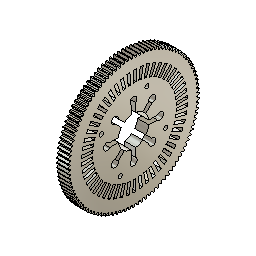
Колесо шестерня v2 (Autodesk Fusion 360 design; units mm, degrees)
Autodesk Fusion 360 part; units mm, degrees
(part 1 of 5)
sketch "Sketch1" plane through (0, 0, 0) normal (1, 0, 0) x (0, 1, 0)
  spline S0 degree 5 poles (13.1929, -43.7407) (13.1941, -43.7421) (13.2057, -43.7558) (13.2278, -43.7819) (13.2606, -43.8203) (13.3041, -43.871) (13.3573, -43.9325) (13.4109, -43.9938) (13.4647, -44.055) (13.5189, -44.116) (13.5735, -44.1768) (13.6283, -44.2375) (13.6834, -44.298) (13.7389, -44.3583) (13.7946, -44.4185) (13.8506, -44.4785) (13.907, -44.5383) (13.9636, -44.5979) (14.0206, -44.6574) (14.0778, -44.7168) (14.1353, -44.7759) (14.1931, -44.8349) (14.2396, -44.882) (14.2745, -44.9172) (14.2979, -44.9406) (14.3096, -44.9524) knots 0.712736 0.712736 0.712736 0.712736 0.712736 0.712736 0.714286 0.728571 0.742857 0.757143 0.771429 0.785714 0.8 0.814286 0.828571 0.842857 0.857143 0.871429 0.885714 0.9 0.914286 0.928571 0.942857 0.957143 0.971429 0.985714 1 1 1 1 1 1
  arc A0 (8.9575, -37.2151) -> (11.0181, -36.7013) centre (0.7975, -0.1016) ccw
  spline S1 degree 5 poles (18.5711, -41.7423) (18.5724, -41.7435) (18.5856, -41.7557) (18.6109, -41.7788) (18.6481, -41.8128) (18.6976, -41.8576) (18.7582, -41.912) (18.819, -41.9661) (18.8801, -42.02) (18.9415, -42.0738) (19.0032, -42.1273) (19.0652, -42.1806) (19.1275, -42.2337) (19.1901, -42.2866) (19.2529, -42.3393) (19.3161, -42.3918) (19.3794, -42.4441) (19.4431, -42.4962) (19.5071, -42.5481) (19.5713, -42.5997) (19.6357, -42.6512) (19.7005, -42.7025) (19.7525, -42.7434) (19.7916, -42.7739) (19.8177, -42.7943) (19.8308, -42.8044) knots 0.712736 0.712736 0.712736 0.712736 0.712736 0.712736 0.714286 0.728571 0.742857 0.757143 0.771429 0.785714 0.8 0.814286 0.828571 0.842857 0.857143 0.871429 0.885714 0.9 0.914286 0.928571 0.942857 0.957143 0.971429 0.985714 1 1 1 1 1 1
  spline S2 degree 5 poles (10.4204, -44.4828) (10.4215, -44.4842) (10.4322, -44.4987) (10.4526, -44.5261) (10.4829, -44.5665) (10.5231, -44.6198) (10.5724, -44.6845) (10.622, -44.7491) (10.6719, -44.8135) (10.7222, -44.8778) (10.7728, -44.9419) (10.8237, -45.0059) (10.8749, -45.0698) (10.9265, -45.1334) (10.9783, -45.197) (11.0305, -45.2604) (11.083, -45.3236) (11.1357, -45.3867) (11.1888, -45.4497) (11.2422, -45.5125) (11.2959, -45.5751) (11.3499, -45.6376) (11.3933, -45.6875) (11.426, -45.7249) (11.4479, -45.7497) (11.4588, -45.7622) knots 0.712736 0.712736 0.712736 0.712736 0.712736 0.712736 0.714286 0.728571 0.742857 0.757143 0.771429 0.785714 0.8 0.814286 0.828571 0.842857 0.857143 0.871429 0.885714 0.9 0.914286 0.928571 0.942857 0.957143 0.971429 0.985714 1 1 1 1 1 1
  spline S3 degree 3 poles (15.9134, -42.826) (15.8674, -42.7781) (15.8125, -42.7397) (15.6911, -42.6859) (15.6257, -42.6712) (15.4929, -42.6676) (15.4268, -42.6788) (15.3026, -42.7258) (15.2457, -42.7613) (15.1487, -42.852) (15.1095, -42.9064) (15.0565, -43.0219) (15.0413, -43.0811) (15.0368, -43.1416) knots 0 0 0 0 0.019923 0.019923 0.039846 0.039846 0.059769 0.059769 0.079691 0.079691 0.099614 0.099614 0.117812 0.117812 0.117812 0.117812
  spline S4 degree 3 poles (13.1929, -43.7407) (13.1501, -43.69) (13.0977, -43.6482) (12.9798, -43.5869) (12.9155, -43.5681) (12.7832, -43.5562) (12.7165, -43.5632) (12.5896, -43.6024) (12.5306, -43.6342) (12.4281, -43.7186) (12.3855, -43.7704) (12.3255, -43.8824) (12.3066, -43.9406) (12.2983, -44.0007) knots 0 0 0 0 0.019923 0.019923 0.039846 0.039846 0.059769 0.059769 0.079691 0.079691 0.099614 0.099614 0.117812 0.117812 0.117812 0.117812
  circle A1 centre (0, 0) radius 11
  circle A2 centre (0, 0) radius 1.5
  spline S5 degree 3 poles (-0.9694, -45.6768) (-0.9945, -45.6153) (-1.0314, -45.5593) (-1.1246, -45.4646) (-1.1799, -45.4268) (-1.3021, -45.3746) (-1.3676, -45.3607) (-1.5004, -45.3587) (-1.5664, -45.3707) (-1.69, -45.4194) (-1.7465, -45.4555) (-1.8382, -45.5434) (-1.8742, -45.5929) (-1.9006, -45.6475) knots 0 0 0 0 0.019923 0.019923 0.039846 0.039846 0.059769 0.059769 0.079691 0.079691 0.099614 0.099614 0.117812 0.117812 0.117812 0.117812
  arc A3 (-0.2495, -30.0833) -> (1.595, -30.091) centre (0.7975, -0.1016) ccw
  spline S6 degree 5 poles (15.9134, -42.826) (15.9146, -42.8273) (15.9271, -42.8403) (15.9508, -42.8649) (15.9859, -42.9012) (16.0325, -42.9491) (16.0895, -43.0071) (16.1468, -43.065) (16.2044, -43.1226) (16.2623, -43.1801) (16.3206, -43.2374) (16.3791, -43.2945) (16.4379, -43.3514) (16.497, -43.4081) (16.5564, -43.4646) (16.6161, -43.521) (16.6761, -43.5772) (16.7364, -43.6332) (16.7969, -43.689) (16.8578, -43.7446) (16.9189, -43.8) (16.9803, -43.8553) (17.0296, -43.8993) (17.0668, -43.9323) (17.0916, -43.9542) (17.104, -43.9652) knots 0.712736 0.712736 0.712736 0.712736 0.712736 0.712736 0.714286 0.728571 0.742857 0.757143 0.771429 0.785714 0.8 0.814286 0.828571 0.842857 0.857143 0.871429 0.885714 0.9 0.914286 0.928571 0.942857 0.957143 0.971429 0.985714 1 1 1 1 1 1
  arc A4 (17.104, -43.9652) -> (17.628, -43.7577) centre (0, 0) ccw
  spline S7 degree 5 poles (17.628, -43.7577) (17.6295, -43.7412) (17.6326, -43.7082) (17.6371, -43.6588) (17.6429, -43.5929) (17.6498, -43.5106) (17.6564, -43.4284) (17.6627, -43.3462) (17.6686, -43.264) (17.6743, -43.182) (17.6795, -43.1) (17.6845, -43.018) (17.6891, -42.9361) (17.6933, -42.8543) (17.6973, -42.7726) (17.7008, -42.6909) (17.7041, -42.6093) (17.707, -42.5277) (17.7095, -42.4462) (17.7117, -42.3648) (17.7135, -42.2835) (17.7147, -42.2168) (17.7154, -42.1663) (17.7158, -42.1321) (17.716, -42.1141) (17.7161, -42.1123) knots -1 -1 -1 -1 -1 -1 -0.985714 -0.971429 -0.957143 -0.942857 -0.928571 -0.914286 -0.9 -0.885714 -0.871429 -0.857143 -0.842857 -0.828571 -0.814286 -0.8 -0.785714 -0.771429 -0.757143 -0.742857 -0.728571 -0.714286 -0.712736 -0.712736 -0.712736 -0.712736 -0.712736 -0.712736
  arc A5 (14.3096, -44.9524) -> (14.8456, -44.7782) centre (0, 0) ccw
  spline S8 degree 5 poles (12.0047, -45.622) (12.0083, -45.6059) (12.0154, -45.5735) (12.0261, -45.525) (12.0401, -45.4604) (12.0573, -45.3796) (12.0742, -45.2989) (12.0907, -45.2181) (12.1069, -45.1374) (12.1228, -45.0566) (12.1383, -44.9759) (12.1534, -44.8953) (12.1683, -44.8146) (12.1828, -44.734) (12.1969, -44.6533) (12.2107, -44.5727) (12.2241, -44.4922) (12.2372, -44.4116) (12.2499, -44.3311) (12.2623, -44.2506) (12.2743, -44.1702) (12.2838, -44.1041) (12.2909, -44.0541) (12.2956, -44.0202) (12.2981, -44.0024) (12.2983, -44.0007) knots -1 -1 -1 -1 -1 -1 -0.985714 -0.971429 -0.957143 -0.942857 -0.928571 -0.914286 -0.9 -0.885714 -0.871429 -0.857143 -0.842857 -0.828571 -0.814286 -0.8 -0.785714 -0.771429 -0.757143 -0.742857 -0.728571 -0.714286 -0.712736 -0.712736 -0.712736 -0.712736 -0.712736 -0.712736
  spline S9 degree 5 poles (14.8456, -44.7782) (14.8482, -44.7619) (14.8533, -44.7291) (14.8609, -44.6801) (14.8709, -44.6147) (14.8829, -44.533) (14.8947, -44.4513) (14.9061, -44.3697) (14.9172, -44.2881) (14.928, -44.2065) (14.9384, -44.125) (14.9485, -44.0436) (14.9582, -43.9621) (14.9676, -43.8807) (14.9766, -43.7994) (14.9853, -43.7181) (14.9937, -43.6368) (15.0017, -43.5556) (15.0093, -43.4745) (15.0166, -43.3934) (15.0235, -43.3123) (15.0289, -43.2458) (15.0328, -43.1954) (15.0354, -43.1613) (15.0367, -43.1434) (15.0368, -43.1416) knots -1 -1 -1 -1 -1 -1 -0.985714 -0.971429 -0.957143 -0.942857 -0.928571 -0.914286 -0.9 -0.885714 -0.871429 -0.857143 -0.842857 -0.828571 -0.814286 -0.8 -0.785714 -0.771429 -0.757143 -0.742857 -0.728571 -0.714286 -0.712736 -0.712736 -0.712736 -0.712736 -0.712736 -0.712736
  spline S10 degree 5 poles (21.1555, -40.4939) (21.1568, -40.495) (21.1708, -40.5063) (21.1974, -40.5278) (21.2368, -40.5594) (21.289, -40.601) (21.3528, -40.6514) (21.4169, -40.7016) (21.4813, -40.7516) (21.546, -40.8014) (21.6109, -40.8509) (21.6762, -40.9002) (21.7417, -40.9493) (21.8074, -40.9982) (21.8734, -41.0468) (21.9397, -41.0953) (22.0063, -41.1435) (22.0731, -41.1915) (22.1402, -41.2392) (22.2075, -41.2868) (22.2751, -41.3341) (22.3429, -41.3812) (22.3974, -41.4188) (22.4383, -41.4468) (22.4657, -41.4655) (22.4794, -41.4748) knots 0.712736 0.712736 0.712736 0.712736 0.712736 0.712736 0.714286 0.728571 0.742857 0.757143 0.771429 0.785714 0.8 0.814286 0.828571 0.842857 0.857143 0.871429 0.885714 0.9 0.914286 0.928571 0.942857 0.957143 0.971429 0.985714 1 1 1 1 1 1
  spline S11 degree 3 poles (21.1555, -40.4939) (21.1038, -40.4521) (21.0445, -40.4208) (20.9173, -40.3827) (20.8506, -40.3763) (20.7184, -40.3894) (20.6542, -40.4087) (20.5369, -40.471) (20.4849, -40.5133) (20.4, -40.6155) (20.3679, -40.6743) (20.3299, -40.7956) (20.3222, -40.8562) (20.3254, -40.9168) knots 0 0 0 0 0.019923 0.019923 0.039846 0.039846 0.059769 0.059769 0.079691 0.079691 0.099614 0.099614 0.117812 0.117812 0.117812 0.117812
  spline S12 degree 3 poles (23.6563, -39.0856) (23.6022, -39.0471) (23.541, -39.0196) (23.4117, -38.9896) (23.3447, -38.9874) (23.2136, -39.0087) (23.1507, -39.0321) (23.0376, -39.1016) (22.9883, -39.1471) (22.91, -39.2544) (22.8817, -39.3152) (22.8514, -39.4386) (22.8475, -39.4996) (22.8544, -39.5598) knots 0 0 0 0 0.019923 0.019923 0.039846 0.039846 0.059769 0.059769 0.079691 0.079691 0.099614 0.099614 0.117812 0.117812 0.117812 0.117812
  spline S13 degree 5 poles (22.9733, -41.2033) (22.9727, -41.1867) (22.9716, -41.1536) (22.9699, -41.104) (22.9674, -41.0379) (22.964, -40.9554) (22.9602, -40.873) (22.9561, -40.7907) (22.9517, -40.7084) (22.947, -40.6263) (22.942, -40.5443) (22.9366, -40.4624) (22.9309, -40.3805) (22.9249, -40.2988) (22.9185, -40.2172) (22.9118, -40.1357) (22.9048, -40.0544) (22.8975, -39.9731) (22.8898, -39.892) (22.8817, -39.8109) (22.8733, -39.73) (22.8662, -39.6636) (22.8606, -39.6135) (22.8567, -39.5795) (22.8546, -39.5616) (22.8544, -39.5598) knots -1 -1 -1 -1 -1 -1 -0.985714 -0.971429 -0.957143 -0.942857 -0.928571 -0.914286 -0.9 -0.885714 -0.871429 -0.857143 -0.842857 -0.828571 -0.814286 -0.8 -0.785714 -0.771429 -0.757143 -0.742857 -0.728571 -0.714286 -0.712736 -0.712736 -0.712736 -0.712736 -0.712736 -0.712736
  spline S14 degree 3 poles (18.5711, -41.7423) (18.5222, -41.6974) (18.465, -41.6624) (18.3404, -41.6164) (18.2742, -41.6058) (18.1414, -41.6106) (18.0762, -41.6259) (17.9552, -41.6807) (17.9006, -41.7196) (17.8095, -41.8162) (17.7738, -41.873) (17.7282, -41.9916) (17.7167, -42.0517) (17.7161, -42.1123) knots 0 0 0 0 0.019923 0.019923 0.039846 0.039846 0.059769 0.059769 0.079691 0.079691 0.099614 0.099614 0.117812 0.117812 0.117812 0.117812
  arc A6 (11.4588, -45.7622) -> (12.0047, -45.622) centre (0, 0) ccw
  spline S15 degree 3 poles (4.7631, -45.4381) (4.7304, -45.3802) (4.6868, -45.3293) (4.5825, -45.2471) (4.5229, -45.2165) (4.3952, -45.18) (4.3283, -45.1744) (4.1963, -45.1891) (4.1324, -45.2093) (4.0159, -45.273) (3.9644, -45.316) (3.8844, -45.4147) (3.8549, -45.4683) (3.8356, -45.5258) knots 0 0 0 0 0.019923 0.019923 0.039846 0.039846 0.059769 0.059769 0.079691 0.079691 0.099614 0.099614 0.117812 0.117812 0.117812 0.117812
  spline S16 degree 5 poles (20.3407, -42.5645) (20.3413, -42.5479) (20.3422, -42.5148) (20.3436, -42.4652) (20.3453, -42.3991) (20.347, -42.3165) (20.3485, -42.234) (20.3496, -42.1516) (20.3504, -42.0693) (20.3508, -41.987) (20.3509, -41.9048) (20.3507, -41.8227) (20.3502, -41.7407) (20.3493, -41.6588) (20.3481, -41.5769) (20.3465, -41.4952) (20.3446, -41.4135) (20.3423, -41.332) (20.3398, -41.2505) (20.3368, -41.1691) (20.3335, -41.0878) (20.3305, -41.0211) (20.3281, -40.9707) (20.3264, -40.9365) (20.3254, -40.9186) (20.3254, -40.9168) knots -1 -1 -1 -1 -1 -1 -0.985714 -0.971429 -0.957143 -0.942857 -0.928571 -0.914286 -0.9 -0.885714 -0.871429 -0.857143 -0.842857 -0.828571 -0.814286 -0.8 -0.785714 -0.771429 -0.757143 -0.742857 -0.728571 -0.714286 -0.712736 -0.712736 -0.712736 -0.712736 -0.712736 -0.712736
  arc A7 (4.2415, -37.9452) -> (6.3503, -37.6937) centre (0.7975, -0.1016) ccw
  arc A8 (19.8308, -42.8044) -> (20.3407, -42.5645) centre (0, 0) ccw
  spline S17 degree 5 poles (-0.9694, -45.6768) (-0.9687, -45.6784) (-0.9619, -45.695) (-0.9489, -45.7267) (-0.9297, -45.7734) (-0.904, -45.835) (-0.8723, -45.9099) (-0.8404, -45.9848) (-0.808, -46.0596) (-0.7753, -46.1344) (-0.7423, -46.2091) (-0.7089, -46.2837) (-0.6751, -46.3583) (-0.641, -46.4328) (-0.6066, -46.5072) (-0.5719, -46.5816) (-0.5368, -46.6559) (-0.5013, -46.7302) (-0.4656, -46.8043) (-0.4295, -46.8784) (-0.3931, -46.9525) (-0.3563, -47.0264) (-0.3267, -47.0856) (-0.3043, -47.1299) (-0.2893, -47.1594) (-0.2818, -47.1742) knots 0.712736 0.712736 0.712736 0.712736 0.712736 0.712736 0.714286 0.728571 0.742857 0.757143 0.771429 0.785714 0.8 0.814286 0.828571 0.842857 0.857143 0.871429 0.885714 0.9 0.914286 0.928571 0.942857 0.957143 0.971429 0.985714 1 1 1 1 1 1
  arc A9 (-0.2818, -47.1742) -> (0.2818, -47.1742) centre (0, 0) ccw
  spline S18 degree 3 poles (10.4204, -44.4828) (10.3808, -44.4295) (10.3311, -44.3845) (10.2174, -44.3159) (10.1543, -44.2931) (10.0231, -44.2729) (9.9561, -44.2757) (9.827, -44.3069) (9.7661, -44.3349) (9.6584, -44.4127) (9.6127, -44.4618) (9.5457, -44.5698) (9.5232, -44.6266) (9.5112, -44.686) knots 0 0 0 0 0.019923 0.019923 0.039846 0.039846 0.059769 0.059769 0.079691 0.079691 0.099614 0.099614 0.117812 0.117812 0.117812 0.117812
  spline S19 degree 5 poles (9.1163, -46.2858) (9.121, -46.2699) (9.1301, -46.2381) (9.1438, -46.1903) (9.1619, -46.1267) (9.1841, -46.0472) (9.206, -45.9676) (9.2276, -45.8881) (9.2488, -45.8085) (9.2697, -45.7289) (9.2903, -45.6494) (9.3105, -45.5698) (9.3303, -45.4902) (9.3498, -45.4106) (9.369, -45.3311) (9.3878, -45.2515) (9.4063, -45.1719) (9.4244, -45.0924) (9.4422, -45.0128) (9.4596, -44.9333) (9.4766, -44.8537) (9.4903, -44.7884) (9.5005, -44.7389) (9.5073, -44.7054) (9.5109, -44.6878) (9.5112, -44.686) knots -1 -1 -1 -1 -1 -1 -0.985714 -0.971429 -0.957143 -0.942857 -0.928571 -0.914286 -0.9 -0.885714 -0.871429 -0.857143 -0.842857 -0.828571 -0.814286 -0.8 -0.785714 -0.771429 -0.757143 -0.742857 -0.728571 -0.714286 -0.712736 -0.712736 -0.712736 -0.712736 -0.712736 -0.712736
  spline S20 degree 3 poles (1.9006, -45.6475) (1.8717, -45.5877) (1.8313, -45.5342) (1.7324, -45.4455) (1.6748, -45.4113) (1.5496, -45.3668) (1.4833, -45.3571) (1.3506, -45.3634) (1.2855, -45.3796) (1.1652, -45.4359) (1.1112, -45.4755) (1.0251, -45.569) (0.9923, -45.6206) (0.9694, -45.6768) knots 0 0 0 0 0.019923 0.019923 0.039846 0.039846 0.059769 0.059769 0.079691 0.079691 0.099614 0.099614 0.117812 0.117812 0.117812 0.117812
  arc A10 (2.6809, -47.0988) -> (3.2433, -47.0634) centre (0, 0) ccw
  spline S21 degree 5 poles (7.6067, -45.0493) (7.6077, -45.0508) (7.6175, -45.0659) (7.6362, -45.0946) (7.6639, -45.1368) (7.7007, -45.1925) (7.7458, -45.2602) (7.7912, -45.3278) (7.837, -45.3952) (7.8831, -45.4625) (7.9296, -45.5297) (7.9764, -45.5967) (8.0235, -45.6637) (8.0709, -45.7305) (8.1187, -45.7971) (8.1668, -45.8637) (8.2152, -45.9301) (8.2639, -45.9964) (8.3129, -46.0625) (8.3623, -46.1286) (8.4119, -46.1945) (8.4619, -46.2602) (8.5021, -46.3128) (8.5324, -46.3521) (8.5526, -46.3783) (8.5628, -46.3914) knots 0.712736 0.712736 0.712736 0.712736 0.712736 0.712736 0.714286 0.728571 0.742857 0.757143 0.771429 0.785714 0.8 0.814286 0.828571 0.842857 0.857143 0.871429 0.885714 0.9 0.914286 0.928571 0.942857 0.957143 0.971429 0.985714 1 1 1 1 1 1
  arc A11 (22.4794, -41.4748) -> (22.9733, -41.2033) centre (0, 0) ccw
  spline S22 degree 5 poles (4.7631, -45.4381) (4.7639, -45.4396) (4.7728, -45.4553) (4.7896, -45.4851) (4.8146, -45.5289) (4.8478, -45.5869) (4.8886, -45.6572) (4.9297, -45.7275) (4.9712, -45.7977) (5.013, -45.8678) (5.0551, -45.9377) (5.0976, -46.0076) (5.1404, -46.0774) (5.1836, -46.147) (5.2271, -46.2165) (5.2709, -46.286) (5.315, -46.3553) (5.3595, -46.4245) (5.4042, -46.4936) (5.4493, -46.5626) (5.4947, -46.6315) (5.5405, -46.7003) (5.5773, -46.7552) (5.6051, -46.7964) (5.6236, -46.8238) (5.6329, -46.8375) knots 0.712736 0.712736 0.712736 0.712736 0.712736 0.712736 0.714286 0.728571 0.742857 0.757143 0.771429 0.785714 0.8 0.814286 0.828571 0.842857 0.857143 0.871429 0.885714 0.9 0.914286 0.928571 0.942857 0.957143 0.971429 0.985714 1 1 1 1 1 1
  arc A12 (-0.5287, -38.0785) -> (1.595, -38.0932) centre (0.7975, -0.1016) ccw
  spline S23 degree 3 poles (7.6067, -45.0493) (7.5705, -44.9937) (7.5238, -44.9456) (7.4146, -44.87) (7.3531, -44.8433) (7.2234, -44.8149) (7.1563, -44.8135) (7.0255, -44.8365) (6.963, -44.8606) (6.8507, -44.9315) (6.802, -44.9776) (6.7283, -45.0812) (6.7023, -45.1365) (6.6866, -45.1951) knots 0 0 0 0 0.019923 0.019923 0.039846 0.039846 0.059769 0.059769 0.079691 0.079691 0.099614 0.099614 0.117812 0.117812 0.117812 0.117812
  arc A13 (8.5628, -46.3914) -> (9.1163, -46.2858) centre (0, 0) ccw
  spline S24 degree 5 poles (1.9006, -45.6475) (1.9013, -45.6491) (1.9092, -45.6653) (1.9241, -45.6961) (1.9463, -45.7414) (1.9758, -45.8013) (2.0121, -45.8741) (2.0487, -45.9468) (2.0857, -46.0195) (2.123, -46.092) (2.1607, -46.1645) (2.1987, -46.2369) (2.2371, -46.3092) (2.2758, -46.3814) (2.3148, -46.4536) (2.3542, -46.5256) (2.3938, -46.5976) (2.4339, -46.6694) (2.4742, -46.7412) (2.5149, -46.8129) (2.5559, -46.8845) (2.5972, -46.956) (2.6305, -47.0132) (2.6556, -47.056) (2.6724, -47.0845) (2.6809, -47.0988) knots 0.712736 0.712736 0.712736 0.712736 0.712736 0.712736 0.714286 0.728571 0.742857 0.757143 0.771429 0.785714 0.8 0.814286 0.828571 0.842857 0.857143 0.871429 0.885714 0.9 0.914286 0.928571 0.942857 0.957143 0.971429 0.985714 1 1 1 1 1 1
  spline S25 degree 5 poles (6.192, -46.7669) (6.1976, -46.7513) (6.2088, -46.7201) (6.2255, -46.6733) (6.2475, -46.611) (6.2747, -46.533) (6.3015, -46.455) (6.328, -46.3769) (6.3542, -46.2988) (6.3801, -46.2207) (6.4056, -46.1426) (6.4307, -46.0645) (6.4556, -45.9863) (6.48, -45.9081) (6.5042, -45.8299) (6.5279, -45.7517) (6.5514, -45.6734) (6.5744, -45.5952) (6.5972, -45.5169) (6.6195, -45.4386) (6.6415, -45.3603) (6.6593, -45.2959) (6.6725, -45.2472) (6.6815, -45.2142) (6.6861, -45.1968) (6.6866, -45.1951) knots -1 -1 -1 -1 -1 -1 -0.985714 -0.971429 -0.957143 -0.942857 -0.928571 -0.914286 -0.9 -0.885714 -0.871429 -0.857143 -0.842857 -0.828571 -0.814286 -0.8 -0.785714 -0.771429 -0.757143 -0.742857 -0.728571 -0.714286 -0.712736 -0.712736 -0.712736 -0.712736 -0.712736 -0.712736
  spline S26 degree 3 poles (-1.9006, 45.6475) (-1.8717, 45.5877) (-1.8313, 45.5342) (-1.7324, 45.4455) (-1.6748, 45.4113) (-1.5496, 45.3668) (-1.4833, 45.3571) (-1.3506, 45.3634) (-1.2855, 45.3796) (-1.1652, 45.4359) (-1.1112, 45.4755) (-1.0251, 45.569) (-0.9923, 45.6206) (-0.9694, 45.6768) knots 0 0 0 0 0.019923 0.019923 0.039846 0.039846 0.059769 0.059769 0.079691 0.079691 0.099614 0.099614 0.117812 0.117812 0.117812 0.117812
  arc A14 (5.6329, -46.8375) -> (6.192, -46.7669) centre (0, 0) ccw
  spline S27 degree 5 poles (3.2433, -47.0634) (3.2499, -47.0482) (3.263, -47.0178) (3.2825, -46.9721) (3.3084, -46.9113) (3.3405, -46.8351) (3.3722, -46.759) (3.4035, -46.6827) (3.4346, -46.6065) (3.4653, -46.5301) (3.4956, -46.4538) (3.5256, -46.3774) (3.5553, -46.3009) (3.5847, -46.2244) (3.6137, -46.1479) (3.6423, -46.0713) (3.6706, -45.9947) (3.6985, -45.918) (3.7261, -45.8413) (3.7533, -45.7646) (3.7802, -45.6878) (3.802, -45.6247) (3.8183, -45.5769) (3.8292, -45.5445) (3.835, -45.5274) (3.8356, -45.5258) knots -1 -1 -1 -1 -1 -1 -0.985714 -0.971429 -0.957143 -0.942857 -0.928571 -0.914286 -0.9 -0.885714 -0.871429 -0.857143 -0.842857 -0.828571 -0.814286 -0.8 -0.785714 -0.771429 -0.757143 -0.742857 -0.728571 -0.714286 -0.712736 -0.712736 -0.712736 -0.712736 -0.712736 -0.712736
  spline S28 degree 5 poles (0.2818, -47.1742) (0.2893, -47.1594) (0.3043, -47.1299) (0.3267, -47.0856) (0.3563, -47.0264) (0.3931, -46.9525) (0.4295, -46.8784) (0.4656, -46.8043) (0.5013, -46.7302) (0.5368, -46.6559) (0.5719, -46.5816) (0.6066, -46.5072) (0.641, -46.4328) (0.6751, -46.3583) (0.7089, -46.2837) (0.7423, -46.2091) (0.7753, -46.1344) (0.808, -46.0596) (0.8404, -45.9848) (0.8723, -45.9099) (0.904, -45.835) (0.9297, -45.7734) (0.9489, -45.7267) (0.9619, -45.695) (0.9687, -45.6784) (0.9694, -45.6768) knots -1 -1 -1 -1 -1 -1 -0.985714 -0.971429 -0.957143 -0.942857 -0.928571 -0.914286 -0.9 -0.885714 -0.871429 -0.857143 -0.842857 -0.828571 -0.814286 -0.8 -0.785714 -0.771429 -0.757143 -0.742857 -0.728571 -0.714286 -0.712736 -0.712736 -0.712736 -0.712736 -0.712736 -0.712736
  arc A15 (3.5165, -29.9781) -> (5.3474, -29.7546) centre (0.7975, -0.1016) ccw
  arc A16 (22.0468, -31.605) -> (23.7736, -30.3687) centre (0.7975, -0.1016) ccw
  line L0 (19.07, -23.8948) -> (23.7736, -30.3687)
  spline S29 degree 3 poles (45.1951, -6.6866) (45.1309, -6.7038) (45.0708, -6.7334) (44.9652, -6.8139) (44.9207, -6.8641) (44.8536, -6.9787) (44.8316, -7.0421) (44.813, -7.1736) (44.8167, -7.2405) (44.8494, -7.3692) (44.8782, -7.4298) (44.9539, -7.5318) (44.9985, -7.5737) (45.0493, -7.6067) knots 0 0 0 0 0.019923 0.019923 0.039846 0.039846 0.059769 0.059769 0.079691 0.079691 0.099614 0.099614 0.117812 0.117812 0.117812 0.117812
  spline S30 degree 3 poles (42.1123, -17.7161) (42.0459, -17.7168) (41.9803, -17.7305) (41.858, -17.7822) (41.8024, -17.8198) (41.7089, -17.9141) (41.6718, -17.97) (41.6211, -18.0927) (41.608, -18.1585) (41.6077, -18.2913) (41.6206, -18.3571) (41.6685, -18.4748) (41.7013, -18.5264) (41.7423, -18.5711) knots 0 0 0 0 0.019923 0.019923 0.039846 0.039846 0.059769 0.059769 0.079691 0.079691 0.099614 0.099614 0.117812 0.117812 0.117812 0.117812
  arc A17 (44.7782, -14.8456) -> (44.9524, -14.3096) centre (0, 0) ccw
  spline S31 degree 5 poles (42.1123, -17.7161) (42.1141, -17.716) (42.1321, -17.7158) (42.1663, -17.7154) (42.2168, -17.7147) (42.2835, -17.7135) (42.3648, -17.7117) (42.4462, -17.7095) (42.5277, -17.707) (42.6093, -17.7041) (42.6909, -17.7008) (42.7726, -17.6973) (42.8543, -17.6933) (42.9361, -17.6891) (43.018, -17.6845) (43.1, -17.6795) (43.182, -17.6743) (43.264, -17.6686) (43.3462, -17.6627) (43.4284, -17.6564) (43.5106, -17.6498) (43.5929, -17.6429) (43.6588, -17.6371) (43.7082, -17.6326) (43.7412, -17.6295) (43.7577, -17.628) knots 0.712736 0.712736 0.712736 0.712736 0.712736 0.712736 0.714286 0.728571 0.742857 0.757143 0.771429 0.785714 0.8 0.814286 0.828571 0.842857 0.857143 0.871429 0.885714 0.9 0.914286 0.928571 0.942857 0.957143 0.971429 0.985714 1 1 1 1 1 1
  spline S32 degree 5 poles (45.5258, -3.8356) (45.5274, -3.835) (45.5445, -3.8292) (45.5769, -3.8183) (45.6247, -3.802) (45.6878, -3.7802) (45.7646, -3.7533) (45.8413, -3.7261) (45.918, -3.6985) (45.9947, -3.6706) (46.0713, -3.6423) (46.1479, -3.6137) (46.2244, -3.5847) (46.3009, -3.5553) (46.3774, -3.5256) (46.4538, -3.4956) (46.5301, -3.4653) (46.6065, -3.4346) (46.6827, -3.4035) (46.759, -3.3722) (46.8351, -3.3405) (46.9113, -3.3084) (46.9721, -3.2825) (47.0178, -3.263) (47.0482, -3.2499) (47.0634, -3.2433) knots 0.712736 0.712736 0.712736 0.712736 0.712736 0.712736 0.714286 0.728571 0.742857 0.757143 0.771429 0.785714 0.8 0.814286 0.828571 0.842857 0.857143 0.871429 0.885714 0.9 0.914286 0.928571 0.942857 0.957143 0.971429 0.985714 1 1 1 1 1 1
  arc A18 (46.2858, -9.1163) -> (46.3914, -8.5628) centre (0, 0) ccw
  spline S33 degree 3 poles (43.1416, -15.0368) (43.0754, -15.0417) (43.0107, -15.0595) (42.8919, -15.1189) (42.8389, -15.1599) (42.7515, -15.2599) (42.718, -15.3179) (42.6751, -15.4436) (42.6661, -15.5101) (42.6741, -15.6426) (42.6911, -15.7075) (42.7464, -15.8219) (42.7823, -15.8714) (42.826, -15.9134) knots 0 0 0 0 0.019923 0.019923 0.039846 0.039846 0.059769 0.059769 0.079691 0.079691 0.099614 0.099614 0.117812 0.117812 0.117812 0.117812
  arc A19 (47.0634, -3.2433) -> (47.0988, -2.6809) centre (0, 0) ccw
  spline S34 degree 5 poles (47.0988, -2.6809) (47.0845, -2.6724) (47.056, -2.6556) (47.0132, -2.6305) (46.956, -2.5972) (46.8845, -2.5559) (46.8129, -2.5149) (46.7412, -2.4742) (46.6694, -2.4339) (46.5976, -2.3938) (46.5256, -2.3542) (46.4536, -2.3148) (46.3814, -2.2758) (46.3092, -2.2371) (46.2369, -2.1987) (46.1645, -2.1607) (46.092, -2.123) (46.0195, -2.0857) (45.9468, -2.0487) (45.8741, -2.0121) (45.8013, -1.9758) (45.7414, -1.9463) (45.6961, -1.9241) (45.6653, -1.9092) (45.6491, -1.9013) (45.6475, -1.9006) knots -1 -1 -1 -1 -1 -1 -0.985714 -0.971429 -0.957143 -0.942857 -0.928571 -0.914286 -0.9 -0.885714 -0.871429 -0.857143 -0.842857 -0.828571 -0.814286 -0.8 -0.785714 -0.771429 -0.757143 -0.742857 -0.728571 -0.714286 -0.712736 -0.712736 -0.712736 -0.712736 -0.712736 -0.712736
  spline S35 degree 5 poles (43.9652, -17.104) (43.9542, -17.0916) (43.9323, -17.0668) (43.8993, -17.0296) (43.8553, -16.9803) (43.8, -16.9189) (43.7446, -16.8578) (43.689, -16.7969) (43.6332, -16.7364) (43.5772, -16.6761) (43.521, -16.6161) (43.4646, -16.5564) (43.4081, -16.497) (43.3514, -16.4379) (43.2945, -16.3791) (43.2374, -16.3206) (43.1801, -16.2623) (43.1226, -16.2044) (43.065, -16.1468) (43.0071, -16.0895) (42.9491, -16.0325) (42.9012, -15.9859) (42.8649, -15.9508) (42.8403, -15.9271) (42.8273, -15.9146) (42.826, -15.9134) knots -1 -1 -1 -1 -1 -1 -0.985714 -0.971429 -0.957143 -0.942857 -0.928571 -0.914286 -0.9 -0.885714 -0.871429 -0.857143 -0.842857 -0.828571 -0.814286 -0.8 -0.785714 -0.771429 -0.757143 -0.742857 -0.728571 -0.714286 -0.712736 -0.712736 -0.712736 -0.712736 -0.712736 -0.712736
  spline S36 degree 5 poles (46.8375, -5.6329) (46.8238, -5.6236) (46.7964, -5.6051) (46.7552, -5.5773) (46.7003, -5.5405) (46.6315, -5.4947) (46.5626, -5.4493) (46.4936, -5.4042) (46.4245, -5.3595) (46.3553, -5.315) (46.286, -5.2709) (46.2165, -5.2271) (46.147, -5.1836) (46.0774, -5.1404) (46.0076, -5.0976) (45.9377, -5.0551) (45.8678, -5.013) (45.7977, -4.9712) (45.7275, -4.9297) (45.6572, -4.8886) (45.5869, -4.8478) (45.5289, -4.8146) (45.4851, -4.7896) (45.4553, -4.7728) (45.4396, -4.7639) (45.4381, -4.7631) knots -1 -1 -1 -1 -1 -1 -0.985714 -0.971429 -0.957143 -0.942857 -0.928571 -0.914286 -0.9 -0.885714 -0.871429 -0.857143 -0.842857 -0.828571 -0.814286 -0.8 -0.785714 -0.771429 -0.757143 -0.742857 -0.728571 -0.714286 -0.712736 -0.712736 -0.712736 -0.712736 -0.712736 -0.712736
  arc A20 (46.7669, -6.192) -> (46.8375, -5.6329) centre (0, 0) ccw
  spline S37 degree 5 poles (45.7622, -11.4588) (45.7497, -11.4479) (45.7249, -11.426) (45.6875, -11.3933) (45.6376, -11.3499) (45.5751, -11.2959) (45.5125, -11.2422) (45.4497, -11.1888) (45.3867, -11.1357) (45.3236, -11.083) (45.2604, -11.0305) (45.197, -10.9783) (45.1334, -10.9265) (45.0698, -10.8749) (45.0059, -10.8237) (44.9419, -10.7728) (44.8778, -10.7222) (44.8135, -10.6719) (44.7491, -10.622) (44.6845, -10.5724) (44.6198, -10.5231) (44.5665, -10.4829) (44.5261, -10.4526) (44.4987, -10.4322) (44.4842, -10.4215) (44.4828, -10.4204) knots -1 -1 -1 -1 -1 -1 -0.985714 -0.971429 -0.957143 -0.942857 -0.928571 -0.914286 -0.9 -0.885714 -0.871429 -0.857143 -0.842857 -0.828571 -0.814286 -0.8 -0.785714 -0.771429 -0.757143 -0.742857 -0.728571 -0.714286 -0.712736 -0.712736 -0.712736 -0.712736 -0.712736 -0.712736
  spline S38 degree 5 poles (44.0007, -12.2983) (44.0024, -12.2981) (44.0202, -12.2956) (44.0541, -12.2909) (44.1041, -12.2838) (44.1702, -12.2743) (44.2506, -12.2623) (44.3311, -12.2499) (44.4116, -12.2372) (44.4922, -12.2241) (44.5727, -12.2107) (44.6533, -12.1969) (44.734, -12.1828) (44.8146, -12.1683) (44.8953, -12.1534) (44.9759, -12.1383) (45.0566, -12.1228) (45.1374, -12.1069) (45.2181, -12.0907) (45.2989, -12.0742) (45.3796, -12.0573) (45.4604, -12.0401) (45.525, -12.0261) (45.5735, -12.0154) (45.6059, -12.0083) (45.622, -12.0047) knots 0.712736 0.712736 0.712736 0.712736 0.712736 0.712736 0.714286 0.728571 0.742857 0.757143 0.771429 0.785714 0.8 0.814286 0.828571 0.842857 0.857143 0.871429 0.885714 0.9 0.914286 0.928571 0.942857 0.957143 0.971429 0.985714 1 1 1 1 1 1
  spline S39 degree 5 poles (44.9524, -14.3096) (44.9406, -14.2979) (44.9172, -14.2745) (44.882, -14.2396) (44.8349, -14.1931) (44.7759, -14.1353) (44.7168, -14.0778) (44.6574, -14.0206) (44.5979, -13.9636) (44.5383, -13.907) (44.4785, -13.8506) (44.4185, -13.7946) (44.3583, -13.7389) (44.298, -13.6834) (44.2375, -13.6283) (44.1768, -13.5735) (44.116, -13.5189) (44.055, -13.4647) (43.9938, -13.4109) (43.9325, -13.3573) (43.871, -13.3041) (43.8203, -13.2606) (43.7819, -13.2278) (43.7558, -13.2057) (43.7421, -13.1941) (43.7407, -13.1929) knots -1 -1 -1 -1 -1 -1 -0.985714 -0.971429 -0.957143 -0.942857 -0.928571 -0.914286 -0.9 -0.885714 -0.871429 -0.857143 -0.842857 -0.828571 -0.814286 -0.8 -0.785714 -0.771429 -0.757143 -0.742857 -0.728571 -0.714286 -0.712736 -0.712736 -0.712736 -0.712736 -0.712736 -0.712736
  spline S40 degree 3 poles (45.6768, -0.9694) (45.6153, -0.9945) (45.5593, -1.0314) (45.4646, -1.1246) (45.4268, -1.1799) (45.3746, -1.3021) (45.3607, -1.3676) (45.3587, -1.5004) (45.3707, -1.5664) (45.4194, -1.69) (45.4555, -1.7465) (45.5434, -1.8382) (45.5929, -1.8742) (45.6475, -1.9006) knots 0 0 0 0 0.019923 0.019923 0.039846 0.039846 0.059769 0.059769 0.079691 0.079691 0.099614 0.099614 0.117812 0.117812 0.117812 0.117812
  spline S41 degree 5 poles (23.6563, -39.0856) (23.6578, -39.0866) (23.6724, -39.097) (23.7004, -39.1168) (23.7416, -39.1459) (23.7964, -39.1841) (23.8632, -39.2305) (23.9304, -39.2765) (23.9978, -39.3224) (24.0654, -39.368) (24.1333, -39.4133) (24.2015, -39.4585) (24.27, -39.5033) (24.3387, -39.548) (24.4076, -39.5924) (24.4768, -39.6366) (24.5463, -39.6805) (24.616, -39.7242) (24.6859, -39.7677) (24.7561, -39.8109) (24.8265, -39.8539) (24.8972, -39.8967) (24.9539, -39.9307) (24.9965, -39.9561) (25.025, -39.973) (25.0393, -39.9814) knots 0.712736 0.712736 0.712736 0.712736 0.712736 0.712736 0.714286 0.728571 0.742857 0.757143 0.771429 0.785714 0.8 0.814286 0.828571 0.842857 0.857143 0.871429 0.885714 0.9 0.914286 0.928571 0.942857 0.957143 0.971429 0.985714 1 1 1 1 1 1
  line L1 (21.908, -21.417) -> (27.3859, -27.2504)
  spline S42 degree 5 poles (44.686, -9.5112) (44.6878, -9.5109) (44.7054, -9.5073) (44.7389, -9.5005) (44.7884, -9.4903) (44.8537, -9.4766) (44.9333, -9.4596) (45.0128, -9.4422) (45.0924, -9.4244) (45.1719, -9.4063) (45.2515, -9.3878) (45.3311, -9.369) (45.4106, -9.3498) (45.4902, -9.3303) (45.5698, -9.3105) (45.6494, -9.2903) (45.7289, -9.2697) (45.8085, -9.2488) (45.8881, -9.2276) (45.9676, -9.206) (46.0472, -9.1841) (46.1267, -9.1619) (46.1903, -9.1438) (46.2381, -9.1301) (46.2699, -9.121) (46.2858, -9.1163) knots 0.712736 0.712736 0.712736 0.712736 0.712736 0.712736 0.714286 0.728571 0.742857 0.757143 0.771429 0.785714 0.8 0.814286 0.828571 0.842857 0.857143 0.871429 0.885714 0.9 0.914286 0.928571 0.942857 0.957143 0.971429 0.985714 1 1 1 1 1 1
  line L2 (23.2315, -20.0194) -> (29.2138, -25.3308)
  spline S43 degree 5 poles (45.1951, -6.6866) (45.1968, -6.6861) (45.2142, -6.6815) (45.2472, -6.6725) (45.2959, -6.6593) (45.3603, -6.6415) (45.4386, -6.6195) (45.5169, -6.5972) (45.5952, -6.5744) (45.6734, -6.5514) (45.7517, -6.5279) (45.8299, -6.5042) (45.9081, -6.48) (45.9863, -6.4556) (46.0645, -6.4307) (46.1426, -6.4056) (46.2207, -6.3801) (46.2988, -6.3542) (46.3769, -6.328) (46.455, -6.3015) (46.533, -6.2747) (46.611, -6.2475) (46.6733, -6.2255) (46.7201, -6.2088) (46.7513, -6.1976) (46.7669, -6.192) knots 0.712736 0.712736 0.712736 0.712736 0.712736 0.712736 0.714286 0.728571 0.742857 0.757143 0.771429 0.785714 0.8 0.814286 0.828571 0.842857 0.857143 0.871429 0.885714 0.9 0.914286 0.928571 0.942857 0.957143 0.971429 0.985714 1 1 1 1 1 1
  arc A21 (43.7577, -17.628) -> (43.9652, -17.104) centre (0, 0) ccw
  line L3 (24.4131, -18.6031) -> (30.5789, -23.7039)
  spline S44 degree 3 poles (44.686, -9.5112) (44.621, -9.5244) (44.5591, -9.5501) (44.4486, -9.6239) (44.4011, -9.6712) (44.3269, -9.7814) (44.301, -9.8432) (44.2742, -9.9732) (44.2736, -10.0403) (44.2982, -10.1708) (44.3231, -10.233) (44.3923, -10.3396) (44.4341, -10.3842) (44.4828, -10.4204) knots 0 0 0 0 0.019923 0.019923 0.039846 0.039846 0.059769 0.059769 0.079691 0.079691 0.099614 0.099614 0.117812 0.117812 0.117812 0.117812
  spline S45 degree 5 poles (46.3914, -8.5628) (46.3783, -8.5526) (46.3521, -8.5324) (46.3128, -8.5021) (46.2602, -8.4619) (46.1945, -8.4119) (46.1286, -8.3623) (46.0625, -8.3129) (45.9964, -8.2639) (45.9301, -8.2152) (45.8637, -8.1668) (45.7971, -8.1187) (45.7305, -8.0709) (45.6637, -8.0235) (45.5967, -7.9764) (45.5297, -7.9296) (45.4625, -7.8831) (45.3952, -7.837) (45.3278, -7.7912) (45.2602, -7.7458) (45.1925, -7.7007) (45.1368, -7.6639) (45.0946, -7.6362) (45.0659, -7.6175) (45.0508, -7.6077) (45.0493, -7.6067) knots -1 -1 -1 -1 -1 -1 -0.985714 -0.971429 -0.957143 -0.942857 -0.928571 -0.914286 -0.9 -0.885714 -0.871429 -0.857143 -0.842857 -0.828571 -0.814286 -0.8 -0.785714 -0.771429 -0.757143 -0.742857 -0.728571 -0.714286 -0.712736 -0.712736 -0.712736 -0.712736 -0.712736 -0.712736
  spline S46 degree 5 poles (42.8044, -19.8308) (42.7943, -19.8177) (42.7739, -19.7916) (42.7434, -19.7525) (42.7025, -19.7005) (42.6512, -19.6357) (42.5997, -19.5713) (42.5481, -19.5071) (42.4962, -19.4431) (42.4441, -19.3794) (42.3918, -19.3161) (42.3393, -19.2529) (42.2866, -19.1901) (42.2337, -19.1275) (42.1806, -19.0652) (42.1273, -19.0032) (42.0738, -18.9415) (42.02, -18.8801) (41.9661, -18.819) (41.912, -18.7582) (41.8576, -18.6976) (41.8128, -18.6481) (41.7788, -18.6109) (41.7557, -18.5856) (41.7435, -18.5724) (41.7423, -18.5711) knots -1 -1 -1 -1 -1 -1 -0.985714 -0.971429 -0.957143 -0.942857 -0.928571 -0.914286 -0.9 -0.885714 -0.871429 -0.857143 -0.842857 -0.828571 -0.814286 -0.8 -0.785714 -0.771429 -0.757143 -0.742857 -0.728571 -0.714286 -0.712736 -0.712736 -0.712736 -0.712736 -0.712736 -0.712736
  line L4 (25.5509, -17.0506) -> (32.1518, -21.5703)
  spline S47 degree 5 poles (43.1416, -15.0368) (43.1434, -15.0367) (43.1613, -15.0354) (43.1954, -15.0328) (43.2458, -15.0289) (43.3123, -15.0235) (43.3934, -15.0166) (43.4745, -15.0093) (43.5556, -15.0017) (43.6368, -14.9937) (43.7181, -14.9853) (43.7994, -14.9766) (43.8807, -14.9676) (43.9621, -14.9582) (44.0436, -14.9485) (44.125, -14.9384) (44.2065, -14.928) (44.2881, -14.9172) (44.3697, -14.9061) (44.4513, -14.8947) (44.533, -14.8829) (44.6147, -14.8709) (44.6801, -14.8609) (44.7291, -14.8533) (44.7619, -14.8482) (44.7782, -14.8456) knots 0.712736 0.712736 0.712736 0.712736 0.712736 0.712736 0.714286 0.728571 0.742857 0.757143 0.771429 0.785714 0.8 0.814286 0.828571 0.842857 0.857143 0.871429 0.885714 0.9 0.914286 0.928571 0.942857 0.957143 0.971429 0.985714 1 1 1 1 1 1
  arc A22 (45.622, -12.0047) -> (45.7622, -11.4588) centre (0, 0) ccw
  spline S48 degree 3 poles (45.5258, -3.8356) (45.4628, -3.8568) (45.4046, -3.8901) (45.3043, -3.9771) (45.2631, -4.03) (45.2033, -4.1486) (45.1853, -4.2132) (45.175, -4.3456) (45.1829, -4.4122) (45.2236, -4.5386) (45.2562, -4.5972) (45.3381, -4.6943) (45.3852, -4.7333) (45.4381, -4.7631) knots 0 0 0 0 0.019923 0.019923 0.039846 0.039846 0.059769 0.059769 0.079691 0.079691 0.099614 0.099614 0.117812 0.117812 0.117812 0.117812
  spline S49 degree 3 poles (44.0007, -12.2983) (43.9349, -12.3073) (43.8715, -12.3291) (43.7566, -12.3958) (43.7062, -12.4401) (43.6253, -12.5454) (43.5955, -12.6054) (43.5606, -12.7336) (43.5558, -12.8004) (43.5721, -12.9322) (43.5931, -12.9959) (43.6555, -13.1066) (43.6944, -13.1538) (43.7407, -13.1929) knots 0 0 0 0 0.019923 0.019923 0.039846 0.039846 0.059769 0.059769 0.079691 0.079691 0.099614 0.099614 0.117812 0.117812 0.117812 0.117812
  line L5 (26.5457, -15.4974) -> (33.3022, -19.7852)
  line L6 (20.5582, -22.674) -> (25.8277, -28.6934)
  line L7 (0.7975, -0.1016) -> (1.183, 10.9362)
  circle A23 centre (9.5671, 23.097) radius 1.5
  line L8 (0, 0) -> (0, 11)
  arc A24 (28.3716, 11.7167) -> (27.5932, 13.3889) centre (0.7975, -0.1016) ccw
  arc A25 (19.2674, 23.5387) -> (17.7796, 24.6291) centre (0.7975, -0.1016) ccw
  arc A26 (26.6729, 15.0794) -> (25.6911, 16.6409) centre (0.7975, -0.1016) ccw
  arc A27 (24.5662, 18.2028) -> (23.3964, 19.6289) centre (0.7975, -0.1016) ccw
  arc A28 (22.0846, 21.0374) -> (20.7453, 22.3057) centre (0.7975, -0.1016) ccw
  spline S50 degree 5 poles (46.7669, 6.192) (46.7513, 6.1976) (46.7201, 6.2088) (46.6733, 6.2255) (46.611, 6.2475) (46.533, 6.2747) (46.455, 6.3015) (46.3769, 6.328) (46.2988, 6.3542) (46.2207, 6.3801) (46.1426, 6.4056) (46.0645, 6.4307) (45.9863, 6.4556) (45.9081, 6.48) (45.8299, 6.5042) (45.7517, 6.5279) (45.6734, 6.5514) (45.5952, 6.5744) (45.5169, 6.5972) (45.4386, 6.6195) (45.3603, 6.6415) (45.2959, 6.6593) (45.2472, 6.6725) (45.2142, 6.6815) (45.1968, 6.6861) (45.1951, 6.6866) knots -1 -1 -1 -1 -1 -1 -0.985714 -0.971429 -0.957143 -0.942857 -0.928571 -0.914286 -0.9 -0.885714 -0.871429 -0.857143 -0.842857 -0.828571 -0.814286 -0.8 -0.785714 -0.771429 -0.757143 -0.742857 -0.728571 -0.714286 -0.712736 -0.712736 -0.712736 -0.712736 -0.712736 -0.712736
  spline S51 degree 5 poles (45.6475, 1.9006) (45.6491, 1.9013) (45.6653, 1.9092) (45.6961, 1.9241) (45.7414, 1.9463) (45.8013, 1.9758) (45.8741, 2.0121) (45.9468, 2.0487) (46.0195, 2.0857) (46.092, 2.123) (46.1645, 2.1607) (46.2369, 2.1987) (46.3092, 2.2371) (46.3814, 2.2758) (46.4536, 2.3148) (46.5256, 2.3542) (46.5976, 2.3938) (46.6694, 2.4339) (46.7412, 2.4742) (46.8129, 2.5149) (46.8845, 2.5559) (46.956, 2.5972) (47.0132, 2.6305) (47.056, 2.6556) (47.0845, 2.6724) (47.0988, 2.6809) knots 0.712736 0.712736 0.712736 0.712736 0.712736 0.712736 0.714286 0.728571 0.742857 0.757143 0.771429 0.785714 0.8 0.814286 0.828571 0.842857 0.857143 0.871429 0.885714 0.9 0.914286 0.928571 0.942857 0.957143 0.971429 0.985714 1 1 1 1 1 1
  arc A29 (30.7858, 0.736) -> (30.6777, 2.5774) centre (0.7975, -0.1016) ccw
  arc A30 (46.8375, 5.6329) -> (46.7669, 6.192) centre (0, 0) ccw
  arc A31 (16.1588, 25.6672) -> (14.5461, 26.5625) centre (0.7975, -0.1016) ccw
  arc A32 (-18.6601, -32.7421) -> (-16.8062, -33.7781) centre (0.7975, -0.1016) ccw
  line L9 (12.808, 27.3893) -> (16.0108, 34.7202)
  line L10 (-19.1503, -22.5089) -> (-24.6282, -28.3422)
  line L11 (-12.9511, -26.7657) -> (-16.8062, -33.7781)
  line L12 (0, 29.8878) -> (0, 37.89)
  line L13 (5.5939, 29.5125) -> (6.873, 37.4096)
  line L14 (-2.1699, -29.9545) -> (-3.1729, -37.8936)
  line L15 (1.8445, 29.8801) -> (2.1237, 37.8752)
  line L16 (-22.8181, 18.3999) -> (-28.9839, 23.5007)
  arc A33 (-29.3095, -23.2871) -> (-27.9672, -24.9329) centre (0.7975, -0.1016) ccw
  arc A34 (5.5939, 29.5125) -> (3.765, 29.7513) centre (0.7975, -0.1016) ccw
  arc A35 (-5.278, -37.6128) -> (-3.1729, -37.8936) centre (0.7975, -0.1016) ccw
  arc A36 (12.808, 27.3893) -> (11.0958, 28.0754) centre (0.7975, -0.1016) ccw
  line L17 (-14.5638, -25.8704) -> (-18.6601, -32.7421)
  line L18 (3.765, 29.7513) -> (4.7679, 37.6904)
  arc A37 (-9.9315, -36.5555) -> (-7.8782, -37.098) centre (0.7975, -0.1016) ccw
  line L19 (14.5461, 26.5625) -> (18.4013, 33.5749)
  arc A38 (-7.6727, -28.881) -> (-5.8881, -29.3472) centre (0.7975, -0.1016) ccw
  arc A39 (2.1237, 37.8752) -> (0, 37.89) centre (0.7975, -0.1016) ccw
  arc A40 (-15.9783, 24.7695) -> (-17.475, 23.6916) centre (0.7975, -0.1016) ccw
  arc A41 (1.8445, 29.8801) -> (0, 29.8878) centre (0.7975, -0.1016) ccw
  line L20 (-16.1846, -24.8323) -> (-20.8882, -31.3062)
  arc A42 (16.0108, 34.7202) -> (14.0417, 35.5157) centre (0.7975, -0.1016) ccw
  arc A43 (9.2678, 28.6778) -> (7.4831, 29.144) centre (0.7975, -0.1016) ccw
  arc A44 (-14.4158, -34.9234) -> (-12.4466, -35.7189) centre (0.7975, -0.1016) ccw
  circle A45 centre (-23.097, 9.5671) radius 1.5
  line L21 (-9.5008, -28.2786) -> (-12.4466, -35.7189)
  spline S52 degree 5 poles (39.0856, 23.6563) (39.0866, 23.6578) (39.097, 23.6724) (39.1168, 23.7004) (39.1459, 23.7416) (39.1841, 23.7964) (39.2305, 23.8632) (39.2765, 23.9304) (39.3224, 23.9978) (39.368, 24.0654) (39.4133, 24.1333) (39.4585, 24.2015) (39.5033, 24.27) (39.548, 24.3387) (39.5924, 24.4076) (39.6366, 24.4768) (39.6805, 24.5463) (39.7242, 24.616) (39.7677, 24.6859) (39.8109, 24.7561) (39.8539, 24.8265) (39.8967, 24.8972) (39.9307, 24.9539) (39.9561, 24.9965) (39.973, 25.025) (39.9814, 25.0393) knots 0.712736 0.712736 0.712736 0.712736 0.712736 0.712736 0.714286 0.728571 0.742857 0.757143 0.771429 0.785714 0.8 0.814286 0.828571 0.842857 0.857143 0.871429 0.885714 0.9 0.914286 0.928571 0.942857 0.957143 0.971429 0.985714 1 1 1 1 1 1
  arc A46 (11.5265, 36.3523) -> (9.4732, 36.8948) centre (0.7975, -0.1016) ccw
  line L22 (-11.213, -27.5925) -> (-14.4158, -34.9234)
  line L23 (-3.9989, -29.7157) -> (-5.278, -37.6128)
  arc A47 (6.873, 37.4096) -> (4.7679, 37.6904) centre (0.7975, -0.1016) ccw
  arc A48 (-3.9989, -29.7157) -> (-2.1699, -29.9545) centre (0.7975, -0.1016) ccw
  arc A49 (-27.3933, 10.159) -> (-27.9705, 8.4072) centre (0.7975, -0.1016) ccw
  line L24 (-5.8881, -29.3472) -> (-7.8782, -37.098)
  line L25 (-17.475, 23.6916) -> (-22.1786, 30.1655)
  line L26 (-28.8101, 4.7345) -> (-36.6706, 6.2339)
  line L27 (-7.6727, -28.881) -> (-9.9315, -36.5555)
  arc A50 (-14.5638, -25.8704) -> (-12.9511, -26.7657) centre (0.7975, -0.1016) ccw
  arc A51 (-33.0003, 17.2681) -> (-33.9179, 15.3528) centre (0.7975, -0.1016) ccw
  line L28 (11.0958, 28.0754) -> (14.0417, 35.5157)
  line L29 (9.2678, 28.6778) -> (11.5265, 36.3523)
  line L30 (-20.313, 21.2138) -> (-25.7909, 27.0472)
  line L31 (-27.9705, 8.4072) -> (-35.5811, 10.88)
  line L32 (7.4831, 29.144) -> (9.4732, 36.8948)
  line L33 (-25.885, 13.6113) -> (-33.0003, 17.2681)
  arc A52 (-27.6188, 25.1276) -> (-28.9839, 23.5007) centre (0.7975, -0.1016) ccw
  line L34 (-26.6773, 11.9457) -> (-33.9179, 15.3528)
  arc A53 (-14.8456, -44.7782) -> (-14.3096, -44.9524) centre (0, 0) ccw
  arc A54 (-28.457, 6.5449) -> (-28.8101, 4.7345) centre (0.7975, -0.1016) ccw
  spline S53 degree 3 poles (-20.3254, -40.9168) (-20.3219, -40.8505) (-20.3314, -40.7841) (-20.3754, -40.6588) (-20.4094, -40.601) (-20.4977, -40.5018) (-20.5511, -40.4613) (-20.6705, -40.403) (-20.7352, -40.3857) (-20.8678, -40.3771) (-20.9343, -40.3858) (-21.0547, -40.4263) (-21.1083, -40.4557) (-21.1555, -40.4939) knots 0 0 0 0 0.019923 0.019923 0.039846 0.039846 0.059769 0.059769 0.079691 0.079691 0.099614 0.099614 0.117812 0.117812 0.117812 0.117812
  arc A55 (-5.6445, 29.1986) -> (-7.433, 28.7473) centre (0.7975, -0.1016) ccw
  line L35 (20.7453, 22.3057) -> (26.2232, 28.139)
  spline S54 degree 5 poles (-39.9814, 25.0393) (-39.973, 25.025) (-39.9561, 24.9965) (-39.9307, 24.9539) (-39.8967, 24.8972) (-39.8539, 24.8265) (-39.8109, 24.7561) (-39.7677, 24.6859) (-39.7242, 24.616) (-39.6805, 24.5463) (-39.6366, 24.4768) (-39.5924, 24.4076) (-39.548, 24.3387) (-39.5033, 24.27) (-39.4585, 24.2015) (-39.4133, 24.1333) (-39.368, 24.0654) (-39.3224, 23.9978) (-39.2765, 23.9304) (-39.2305, 23.8632) (-39.1841, 23.7964) (-39.1459, 23.7416) (-39.1168, 23.7004) (-39.097, 23.6724) (-39.0866, 23.6578) (-39.0856, 23.6563) knots -1 -1 -1 -1 -1 -1 -0.985714 -0.971429 -0.957143 -0.942857 -0.928571 -0.914286 -0.9 -0.885714 -0.871429 -0.857143 -0.842857 -0.828571 -0.814286 -0.8 -0.785714 -0.771429 -0.757143 -0.742857 -0.728571 -0.714286 -0.712736 -0.712736 -0.712736 -0.712736 -0.712736 -0.712736
  line L36 (-23.9559, 16.8474) -> (-30.5568, 21.3671)
  arc A56 (-29.0593, 2.8259) -> (-29.1828, 0.9855) centre (0.7975, -0.1016) ccw
  arc A57 (20.2551, 32.5389) -> (18.4013, 33.5749) centre (0.7975, -0.1016) ccw
  arc A58 (3.2433, 47.0634) -> (2.6809, 47.0988) centre (0, 0) ccw
  arc A59 (-3.2433, -47.0634) -> (-2.6809, -47.0988) centre (0, 0) ccw
  spline S55 degree 3 poles (-12.2983, -44.0007) (-12.3073, -43.9349) (-12.3291, -43.8715) (-12.3958, -43.7566) (-12.4401, -43.7062) (-12.5454, -43.6253) (-12.6054, -43.5955) (-12.7336, -43.5606) (-12.8004, -43.5558) (-12.9322, -43.5721) (-12.9959, -43.5931) (-13.1066, -43.6555) (-13.1538, -43.6944) (-13.1929, -43.7407) knots 0 0 0 0 0.019923 0.019923 0.039846 0.039846 0.059769 0.059769 0.079691 0.079691 0.099614 0.099614 0.117812 0.117812 0.117812 0.117812
  spline S56 degree 5 poles (5.6329, 46.8375) (5.6236, 46.8238) (5.6051, 46.7964) (5.5773, 46.7552) (5.5405, 46.7003) (5.4947, 46.6315) (5.4493, 46.5626) (5.4042, 46.4936) (5.3595, 46.4245) (5.315, 46.3553) (5.2709, 46.286) (5.2271, 46.2165) (5.1836, 46.147) (5.1404, 46.0774) (5.0976, 46.0076) (5.0551, 45.9377) (5.013, 45.8678) (4.9712, 45.7977) (4.9297, 45.7275) (4.8886, 45.6572) (4.8478, 45.5869) (4.8146, 45.5289) (4.7896, 45.4851) (4.7728, 45.4553) (4.7639, 45.4396) (4.7631, 45.4381) knots -1 -1 -1 -1 -1 -1 -0.985714 -0.971429 -0.957143 -0.942857 -0.928571 -0.914286 -0.9 -0.885714 -0.871429 -0.857143 -0.842857 -0.828571 -0.814286 -0.8 -0.785714 -0.771429 -0.757143 -0.742857 -0.728571 -0.714286 -0.712736 -0.712736 -0.712736 -0.712736 -0.712736 -0.712736
  line L37 (-3.7524, 29.5514) -> (-4.7553, 37.4905)
  spline S57 degree 5 poles (-3.8356, -45.5258) (-3.835, -45.5274) (-3.8292, -45.5445) (-3.8183, -45.5769) (-3.802, -45.6247) (-3.7802, -45.6878) (-3.7533, -45.7646) (-3.7261, -45.8413) (-3.6985, -45.918) (-3.6706, -45.9947) (-3.6423, -46.0713) (-3.6137, -46.1479) (-3.5847, -46.2244) (-3.5553, -46.3009) (-3.5256, -46.3774) (-3.4956, -46.4538) (-3.4653, -46.5301) (-3.4346, -46.6065) (-3.4035, -46.6827) (-3.3722, -46.759) (-3.3405, -46.8351) (-3.3084, -46.9113) (-3.2825, -46.9721) (-3.263, -47.0178) (-3.2499, -47.0482) (-3.2433, -47.0634) knots 0.712736 0.712736 0.712736 0.712736 0.712736 0.712736 0.714286 0.728571 0.742857 0.757143 0.771429 0.785714 0.8 0.814286 0.828571 0.842857 0.857143 0.871429 0.885714 0.9 0.914286 0.928571 0.942857 0.957143 0.971429 0.985714 1 1 1 1 1 1
  arc A60 (6.192, 46.7669) -> (5.6329, 46.8375) centre (0, 0) ccw
  line L38 (19.2674, 23.5387) -> (24.1926, 29.8428)
  spline S58 degree 5 poles (-14.3096, -44.9524) (-14.2979, -44.9406) (-14.2745, -44.9172) (-14.2396, -44.882) (-14.1931, -44.8349) (-14.1353, -44.7759) (-14.0778, -44.7168) (-14.0206, -44.6574) (-13.9636, -44.5979) (-13.907, -44.5383) (-13.8506, -44.4785) (-13.7946, -44.4185) (-13.7389, -44.3583) (-13.6834, -44.298) (-13.6283, -44.2375) (-13.5735, -44.1768) (-13.5189, -44.116) (-13.4647, -44.055) (-13.4109, -43.9938) (-13.3573, -43.9325) (-13.3041, -43.871) (-13.2606, -43.8203) (-13.2278, -43.7819) (-13.2057, -43.7558) (-13.1941, -43.7421) (-13.1929, -43.7407) knots -1 -1 -1 -1 -1 -1 -0.985714 -0.971429 -0.957143 -0.942857 -0.928571 -0.914286 -0.9 -0.885714 -0.871429 -0.857143 -0.842857 -0.828571 -0.814286 -0.8 -0.785714 -0.771429 -0.757143 -0.742857 -0.728571 -0.714286 -0.712736 -0.712736 -0.712736 -0.712736 -0.712736 -0.712736
  spline S59 degree 5 poles (14.3096, 44.9524) (14.2979, 44.9406) (14.2745, 44.9172) (14.2396, 44.882) (14.1931, 44.8349) (14.1353, 44.7759) (14.0778, 44.7168) (14.0206, 44.6574) (13.9636, 44.5979) (13.907, 44.5383) (13.8506, 44.4785) (13.7946, 44.4185) (13.7389, 44.3583) (13.6834, 44.298) (13.6283, 44.2375) (13.5735, 44.1768) (13.5189, 44.116) (13.4647, 44.055) (13.4109, 43.9938) (13.3573, 43.9325) (13.3041, 43.871) (13.2606, 43.8203) (13.2278, 43.7819) (13.2057, 43.7558) (13.1941, 43.7421) (13.1929, 43.7407) knots -1 -1 -1 -1 -1 -1 -0.985714 -0.971429 -0.957143 -0.942857 -0.928571 -0.914286 -0.9 -0.885714 -0.871429 -0.857143 -0.842857 -0.828571 -0.814286 -0.8 -0.785714 -0.771429 -0.757143 -0.742857 -0.728571 -0.714286 -0.712736 -0.712736 -0.712736 -0.712736 -0.712736 -0.712736
  spline S60 degree 3 poles (-9.5112, -44.686) (-9.5244, -44.621) (-9.5501, -44.5591) (-9.6239, -44.4486) (-9.6712, -44.4011) (-9.7814, -44.3269) (-9.8432, -44.301) (-9.9732, -44.2742) (-10.0403, -44.2736) (-10.1708, -44.2982) (-10.233, -44.3231) (-10.3396, -44.3923) (-10.3842, -44.4341) (-10.4204, -44.4828) knots 0 0 0 0 0.019923 0.019923 0.039846 0.039846 0.059769 0.059769 0.079691 0.079691 0.099614 0.099614 0.117812 0.117812 0.117812 0.117812
  arc A61 (-18.9632, 22.4708) -> (-20.313, 21.2138) centre (0.7975, -0.1016) ccw
  spline S61 degree 5 poles (-2.6809, -47.0988) (-2.6724, -47.0845) (-2.6556, -47.056) (-2.6305, -47.0132) (-2.5972, -46.956) (-2.5559, -46.8845) (-2.5149, -46.8129) (-2.4742, -46.7412) (-2.4339, -46.6694) (-2.3938, -46.5976) (-2.3542, -46.5256) (-2.3148, -46.4536) (-2.2758, -46.3814) (-2.2371, -46.3092) (-2.1987, -46.2369) (-2.1607, -46.1645) (-2.123, -46.092) (-2.0857, -46.0195) (-2.0487, -45.9468) (-2.0121, -45.8741) (-1.9758, -45.8013) (-1.9463, -45.7414) (-1.9241, -45.6961) (-1.9092, -45.6653) (-1.9013, -45.6491) (-1.9006, -45.6475) knots -1 -1 -1 -1 -1 -1 -0.985714 -0.971429 -0.957143 -0.942857 -0.928571 -0.914286 -0.9 -0.885714 -0.871429 -0.857143 -0.842857 -0.828571 -0.814286 -0.8 -0.785714 -0.771429 -0.757143 -0.742857 -0.728571 -0.714286 -0.712736 -0.712736 -0.712736 -0.712736 -0.712736 -0.712736
  arc A62 (0.2818, 47.1742) -> (-0.2818, 47.1742) centre (0, 0) ccw
  line L39 (-15.9783, 24.7695) -> (-20.4518, 31.4018)
  line L40 (-5.6445, 29.1986) -> (-7.3624, 37.0119)
  line L41 (-14.3489, 25.7941) -> (-18.204, 32.8065)
  line L42 (-28.457, 6.5449) -> (-36.2582, 8.3172)
  spline S62 degree 5 poles (-11.4588, -45.7622) (-11.4479, -45.7497) (-11.426, -45.7249) (-11.3933, -45.6875) (-11.3499, -45.6376) (-11.2959, -45.5751) (-11.2422, -45.5125) (-11.1888, -45.4497) (-11.1357, -45.3867) (-11.083, -45.3236) (-11.0305, -45.2604) (-10.9783, -45.197) (-10.9265, -45.1334) (-10.8749, -45.0698) (-10.8237, -45.0059) (-10.7728, -44.9419) (-10.7222, -44.8778) (-10.6719, -44.8135) (-10.622, -44.7491) (-10.5724, -44.6845) (-10.5231, -44.6198) (-10.4829, -44.5665) (-10.4526, -44.5261) (-10.4322, -44.4987) (-10.4215, -44.4842) (-10.4204, -44.4828) knots -1 -1 -1 -1 -1 -1 -0.985714 -0.971429 -0.957143 -0.942857 -0.928571 -0.914286 -0.9 -0.885714 -0.871429 -0.857143 -0.842857 -0.828571 -0.814286 -0.8 -0.785714 -0.771429 -0.757143 -0.742857 -0.728571 -0.714286 -0.712736 -0.712736 -0.712736 -0.712736 -0.712736 -0.712736